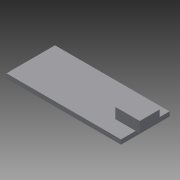
# Autodesk Inventor part: ArduinoNano
Saved by Autodesk Inventor 2014 SP1 (Build 180222100, 222)
## iProperties
Created: 2017-05-21
Part Number: ArduinoNano
Material: Generic
Document SubType Name: Modeling
Designer: danielsikar
Density: 1 g/cm^3
Appearance: Default
Author: danielsikar
Autodesk Inventor part; units mm, degrees
ref_plane "YZ Plane" through (0, 0, 0) normal (1, 0, 0) x (0, 1, 0)
ref_plane "XZ Plane" through (0, 0, 0) normal (0, 1, 0) x (-1, 0, 0)
ref_plane "XY Plane" through (0, 0, 0) normal (0, 0, 1) x (1, 0, 0)
sketch "Sketch1" plane through (0, 0, 0) normal (0, 0, 1) x (1, 0, 0)
  line L0 (0, 0) -> (43.3, 0)
  line L1 (43.3, 0) -> (43.3, 18.36)
  line L2 (43.3, 18.36) -> (0, 18.36)
  line L3 (0, 18.36) -> (0, 0)
  dimension "d0" = 43.3
  dimension "d1" = 18.36
  constraints: 8 end point, 2 parallel, 1 horizontal, 1 perpendicular
  measures "d0" distance of L2.end L1.end
  measures "d1" distance between parallel lines of L0 L2
extrude "Extrusion1" add sketch "Sketch1" along normal blind 1.7
sketch "Sketch2" plane through (0, 0, 1.7) normal (0, 0, 1) x (1, 0, 0)
  line L0 (43.3, 0) -> (43.3, 18.36) projected
  line L1 (43.3, 18.36) -> (0, 18.36) projected
  line L2 (35.62, 13.16) -> (44.82, 13.16)
  line L3 (44.82, 13.16) -> (44.82, 5.58)
  line L4 (44.82, 5.58) -> (35.62, 5.58)
  line L5 (35.62, 5.58) -> (35.62, 13.16)
  dimension "d4" = 9.2
  dimension "d5" = 7.58
  dimension "d6" = 5.2
  dimension "d7" = 1.52
  constraints: 8 end point, 2 parallel, 1 horizontal, 1 perpendicular
  measures "d4" distance of L3.end L4.end
  measures "d5" distance of L2.end L3.end
  measures "d6" distance between parallel lines of L2 L1
  measures "d7" distance between parallel lines of L3 L0
extrude "Extrusion2" add sketch "Sketch2" along normal blind 4
body "Solid1"
